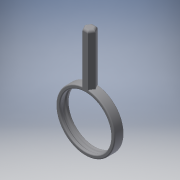
# Autodesk Inventor part: Magnifier Glass Holder
Saved by Autodesk Inventor 2016 (Build 200138000, 138)
## iProperties
Created: 2014-08-03
Part Number: Magnifier Glass Holder
Material: Generic
Document SubType Name: Modeling
Designer: steele
Density: 1 g/cm^3
Appearance: Default
Author: steele
Autodesk Inventor part; units mm, degrees
ref_plane "YZ Plane" through (0, 0, 0) normal (1, 0, 0) x (0, 1, 0)
ref_plane "XZ Plane" through (0, 0, 0) normal (0, 1, 0) x (-1, 0, 0)
sketch "Sketch1" plane through (0, 0, 0) normal (0, 0, 1) x (1, 0, 0)
  line L0 (0, 0) -> (50, 0) construction
  line L1 (50, 0) -> (50, 2)
  line L2 (55, 0) -> (55, 9)
  line L3 (55, 9) -> (48, 9)
  line L4 (48, 9) -> (48, 4)
  line L5 (48, 4) -> (50, 2)
  line L6 (50, 0) -> (55, 0) construction
  line L7 (50, 0) -> (50, -2)
  line L8 (55, 0) -> (55, -9)
  line L9 (55, -9) -> (48, -9)
  line L10 (48, -9) -> (48, -4)
  line L11 (48, -4) -> (50, -2)
  line L12 (0, -12.6) -> (0, 12.6) projected
  dimension "d0" = 50
  dimension "d1" = 9
  dimension "d2" = 5
  dimension "d3" = 7
  dimension "d4" = 5
  constraints: 24 end point, 4 symmetric about line, 3 perpendicular, 1 horizontal, 1 parallel
  measures "d0" distance of L0.start L0.end
  measures "d1" distance of L2.start L2.end
  measures "d2" distance between parallel lines of L1 L2
  measures "d3" distance of L2.end L3.end
  measures "d4" distance of L3.end L4.end
revolve "Revolution1" add sketch "Sketch1" angle 360 about axis through (0, -10, 0) along (0, 1, 0)
ref_plane "Work Plane1" through (0, 0, 50) normal (0, 0, 1) x (1, 0, 0)
sketch "Sketch2" plane through (0, 0, 50) normal (0, 0, 1) x (1, 0, 0)
  line L0 (10.3923, 0) -> (5.1962, -9)
  line L1 (5.1962, -9) -> (-5.1962, -9)
  line L2 (-5.1962, -9) -> (-10.3923, 0)
  line L3 (-10.3923, 0) -> (-5.1962, 9)
  line L4 (-5.1962, 9) -> (5.1962, 9)
  line L5 (5.1962, 9) -> (10.3923, 0)
  point P0 (0, 0)
  point P1 (0, 0)
  dimension "d15" = 18
  constraints: 12 end point, 1 coincident, 13 other
  measures "d15" distance between parallel lines of L1 L4
extrude "Extrusion1" add sketch "Sketch2" along normal blind 100
fillet "Fillet2" radius 2 2 edges at (0, 9, -55) (0, -9, -55)
fillet "Fillet3" [suppressed]
fillet "Fillet4" radius 2 2 edges at (-48, -9, 0) (-48, 9, 0)
fillet "Fillet5" radius 1 4 edges at (-48, -4, 0) (-50, -2, 0) (-48, 4, 0) (-50, 2, 0)
fillet "Fillet6" radius 4.5 6 edges at (0, -9, 150) (7.7942, -4.5, 150) (7.7942, 4.5, 150) (0, 9, 150) (-7.7942, 4.5, 150) (-7.7942, -4.5, 150)
body "Solid1"
